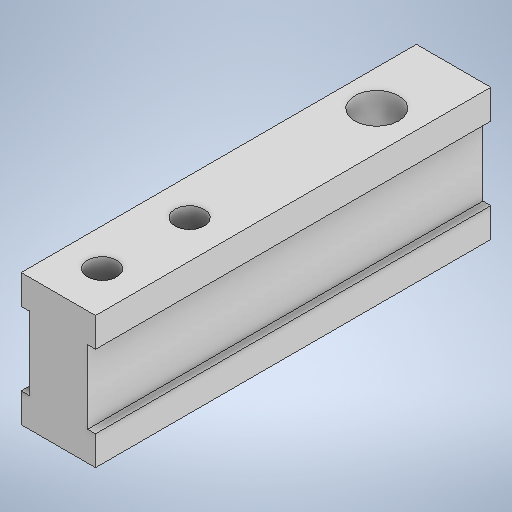
# Autodesk Inventor part: UpperGripperfingerpart
Saved by Autodesk Inventor 2025.1 (Build 291241000, 241)
## iProperties
Created: 2025-02-25
Part Number: UpperGripperfingerpart
Material: Generic
Document SubType Name: Modeling
Designer: m_kni
Density: 1 g/cm^3
Appearance: Default
Author: m_kni
Autodesk Inventor part; units mm, degrees
ref_plane "YZ Plane" through (0, 0, 0) normal (1, 0, 0) x (0, 1, 0)
ref_plane "XZ Plane" through (0, 0, 0) normal (0, 1, 0) x (-1, 0, 0)
ref_plane "XY Plane" through (0, 0, 0) normal (0, 0, 1) x (1, 0, 0)
sketch "Sketch1" plane through (0, 0, 0) normal (0, 0, 1) x (1, 0, 0)
  line L0 (2.1107, -2.6582) -> (2.6507, -2.6582)
  line L1 (2.6507, 2.3418) -> (2.1107, 2.3418)
  line L2 (-1.8893, -2.6582) -> (-1.8893, 2.3418)
  line L3 (-2.4293, -2.6582) -> (-1.8893, -2.6582)
  line L4 (-1.8893, 2.3418) -> (-2.4293, 2.3418)
  line L5 (2.6507, -4.6582) -> (2.6507, -2.6582)
  line L6 (2.6507, -4.6582) -> (1.9068, -4.6582)
  line L7 (0.1107, 4.3418) -> (-1.6853, 4.3418)
  line L8 (-2.4293, 2.3418) -> (-2.4293, 4.3418)
  line L9 (-1.6853, 4.3418) -> (-2.4293, 4.3418)
  line L10 (2.6507, -4.6582) -> (1.9068, -4.6582)
  line L11 (1.9068, -4.6582) -> (1.9068, 4.3418)
  line L12 (2.6507, 4.3418) -> (1.9068, 4.3418)
  line L13 (2.6507, 2.3418) -> (2.6507, 4.3418)
  line L14 (2.6507, 2.3418) -> (2.1107, 2.3418)
  line L15 (2.1107, 2.3418) -> (2.1107, -2.6582)
  line L16 (2.1107, -2.6582) -> (2.6507, -2.6582)
  line L17 (2.6507, -4.6582) -> (2.6507, -2.6582)
  line L18 (-1.6853, -4.6582) -> (-1.6853, 4.3418)
  line L19 (-1.6853, -4.6582) -> (-2.4293, -4.6582)
  line L20 (-2.4293, -4.6582) -> (-2.4293, -2.6582)
  line L21 (-2.4293, -2.6582) -> (-1.8893, -2.6582)
  line L22 (-1.8893, -2.6582) -> (-1.8893, 2.3418)
  line L23 (-1.8893, 2.3418) -> (-2.4293, 2.3418)
  line L24 (-2.4293, 2.3418) -> (-2.4293, 4.3418)
  line L25 (-1.6853, 4.3418) -> (-2.4293, 4.3418)
  line L26 (-1.6853, -4.6582) -> (-1.6853, 4.3418)
  line L27 (2.6507, -4.6582) -> (-2.4293, -4.6582)
  line L28 (2.1107, 2.3418) -> (2.1107, -2.6582)
  line L29 (-1.6853, -4.6582) -> (-2.4293, -4.6582)
  line L30 (2.6507, -4.6582) -> (-2.4293, -4.6582)
  line L31 (2.6507, -2.6582) -> (2.1107, -2.6582)
  line L32 (2.1107, -2.6582) -> (2.1107, 2.3418)
  line L33 (2.1107, 2.3418) -> (2.6507, 2.3418)
  line L34 (2.6507, 2.3418) -> (2.6507, 4.3418)
  line L35 (-2.4293, 4.3418) -> (2.6507, 4.3418)
  line L36 (-2.4293, 2.3418) -> (-2.4293, 4.3418)
  line L37 (-2.4293, 2.3418) -> (-1.8893, 2.3418)
  line L38 (-1.8893, 2.3418) -> (-1.8893, -2.6582)
  line L39 (-1.8893, -2.6582) -> (-2.4293, -2.6582)
  line L40 (-2.4293, -4.6582) -> (-2.4293, -2.6582)
  line L41 (2.6507, -4.6582) -> (-2.4293, -4.6582)
  line L42 (2.6507, -2.6582) -> (2.6507, -4.6582)
  line L43 (-1.3893, 4.3418) -> (1.6107, 4.3418)
  line L44 (1.9068, 4.3418) -> (0.1107, 4.3418)
  line L45 (0.1107, 4.3418) -> (-1.6853, 4.3418)
  line L46 (-1.6853, 4.3418) -> (-2.4293, 4.3418)
  line L47 (-2.4293, 4.3418) -> (2.6507, 4.3418)
  line L48 (2.6507, 4.3418) -> (1.9068, 4.3418)
  line L49 (2.6507, -4.6582) -> (-2.4293, -4.6582)
  line L50 (2.6507, -4.6582) -> (-2.4293, -4.6582)
  line L51 (2.6507, 2.3418) -> (2.6507, 4.3418)
  line L52 (2.1107, 2.3418) -> (2.6507, 2.3418)
  line L53 (2.6507, 2.3418) -> (2.6507, 4.3418)
  line L54 (2.6507, -2.6582) -> (2.1107, -2.6582)
  line L55 (2.6507, 2.3418) -> (2.6507, 4.3418)
  line L56 (2.6507, 2.3418) -> (2.6507, 4.3418)
  line L57 (2.6507, -2.6582) -> (2.6507, -4.6582)
  line L58 (2.6507, -4.6582) -> (2.6507, -2.6582)
  line L59 (2.6507, 2.3418) -> (2.1107, 2.3418)
  line L60 (2.1107, 2.3418) -> (2.6507, 2.3418)
  line L61 (2.1107, -2.6582) -> (2.6507, -2.6582)
  line L62 (2.6507, -2.6582) -> (2.1107, -2.6582)
  line L63 (2.1107, 2.3418) -> (2.1107, -2.6582)
  line L64 (2.1107, -2.6582) -> (2.1107, 2.3418)
  line L65 (-2.4293, -4.6582) -> (-2.4293, -2.6582)
  line L66 (2.6507, 4.3418) -> (1.9068, 4.3418)
  line L67 (-2.4293, 2.3418) -> (-2.4293, 4.3418)
  line L68 (-2.4293, -4.6582) -> (-2.4293, -2.6582)
  line L69 (-1.8893, -2.6582) -> (-2.4293, -2.6582)
  line L70 (-2.4293, 2.3418) -> (-1.8893, 2.3418)
  line L71 (-1.8893, -2.6582) -> (-1.8893, 2.3418)
  line L72 (-1.8893, 2.3418) -> (-1.8893, -2.6582)
  line L73 (-1.8893, -2.6582) -> (-2.4293, -2.6582)
  line L74 (-2.4293, -2.6582) -> (-1.8893, -2.6582)
  line L75 (-1.8893, 2.3418) -> (-2.4293, 2.3418)
  line L76 (-2.4293, 2.3418) -> (-1.8893, 2.3418)
  line L77 (-2.4293, -4.6582) -> (-2.4293, -2.6582)
  line L78 (-2.4293, -4.6582) -> (-2.4293, -2.6582)
  line L79 (-2.4293, 2.3418) -> (-2.4293, 4.3418)
  line L80 (-2.4293, 2.3418) -> (-2.4293, 4.3418)
  line L81 (-2.4293, 4.3418) -> (2.6507, 4.3418)
  line L82 (-1.8893, 2.3418) -> (-1.8893, -2.6582)
  line L83 (2.6507, -2.6582) -> (2.6507, -4.6582)
  line L84 (1.9068, -4.6582) -> (1.9068, 4.3418)
  line L85 (-1.3893, -3.6582) -> (1.6107, -3.6582)
  line L86 (-1.3893, -3.6582) -> (1.6107, -3.6582)
  line L87 (-1.3893, 4.3418) -> (1.6107, 4.3418)
  line L88 (-1.3893, -3.6582) -> (1.6107, -3.6582)
  line L89 (-1.3893, 4.3418) -> (1.6107, 4.3418)
  line L90 (2.1107, -2.6582) -> (2.1107, 2.3418)
  line L91 (1.9068, 4.3418) -> (0.1107, 4.3418)
  line L92 (2.6507, 2.8418) -> (-2.4293, 2.8418)
  line L93 (2.6507, 2.8418) -> (-2.4293, 2.8418)
  line L94 (-2.4293, 2.8418) -> (2.6507, 2.8418)
  line L95 (2.6507, 2.8418) -> (-2.4293, 2.8418)
  point P0 (0, 0)
  point P1 (0.1107, 2.8418)
  point P2 (0.1107, 2.8418)
  point P3 (0.1107, 2.8418)
  point P4 (-2.4293, 2.8418)
  point P5 (2.6507, 2.8418)
  point P6 (2.6507, 2.8418)
  point P7 (0.1107, 2.8418)
  point P8 (0.1107, 2.8418)
  point P9 (0.1107, 2.8418)
  point P10 (0.1107, 2.8418)
  constraints: 176 end point, 24 other
extrude "Extrusion1" add sketch "Sketch1" along normal blind 27
sketch "Sketch2" plane through (-2.4293, 4.3418, 0) normal (0, 1, 0) x (1, 0, 0)
  line L0 (0, -27) -> (5.08, -27) projected
  circle A0 centre (2.4293, -5.14) radius 1.5
  point P0 (2.4293, 0)
  point P1 (2.54, -27)
  point P2 (2.4293, 0)
  dimension "d2" = 21.86
  dimension "d3" = 3
  constraints: 2 coincident, 1 centre point, 1 midpoint
  measures "d2" distance from line of point (2.429, -5.14) L0
  measures "d3" diameter of A0
extrude "Extrusion2" cut sketch "Sketch2" against normal blind 27
sketch "Sketch3" plane through (-2.4293, -4.6582, 0) normal (0, -1, 0) x (1, 0, 0)
  line L0 (5.08, 27) -> (0, 27) projected
  line L1 (2.54, 27) -> (2.4293, 0)
  circle A0 centre (2.5277, 24) radius 1
  circle A1 centre (2.5031, 18) radius 1
  dimension "d6" = 2
  dimension "d7" = 2
  dimension "d8" = 3
  dimension "d9" = 9
  dimension "d10" = 5.08
  constraints: 2 centre point, 2 coincident, 2 end point, 2 point on line, 1 midpoint
  measures "d6" diameter of A0
  measures "d7" diameter of A1
  measures "d8" distance from line of A0.centre L0
  measures "d9" distance from line of A1.centre L0
  measures "d10" distance of L0.end L0.start
extrude "Extrusion3" cut sketch "Sketch3" against normal blind 27
body "Solid1"
